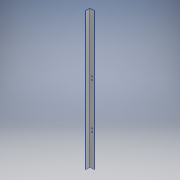
# Autodesk Inventor part: 1400-06-04 Profilé vertical chaniere
Saved by Autodesk Inventor 2017 (Build 210142000, 142)
## iProperties
Part Number: 1400-06-04 Profilé vertical chaniere
Project: 1400-PopCorn Machine
Material: Aluminium 6061
Catalog Web Link: http://www.frenchmakers.com/
Document SubType Name: Modeling
Designer: FABLAB Frenchmakers
Density: 2.7 g/cm^3
Appearance: Aluminium - Plat
Stock Number: 1400-06-03
RuleStatus: InUse
Company: FABLAB Frenchmakers
Author: Adrien MARY
Autodesk Inventor part; units mm, degrees
ref_plane "YZ Plane" through (0, 0, 0) normal (1, 0, 0) x (0, 1, 0)
ref_plane "XZ Plane" through (0, 0, 0) normal (0, 1, 0) x (-1, 0, 0)
ref_plane "XY Plane" through (0, 0, 0) normal (0, 0, 1) x (1, 0, 0)
sketch "Esquisse1" plane through (0, 0, 0) normal (0, 0, 1) x (1, 0, 0)
  line L0 (0, 0) -> (18.3, 0)
  line L1 (18.3, 0) -> (18.3, 2.2)
  line L2 (18.3, 2.2) -> (-2.2, 2.2)
  line L3 (-2.2, 2.2) -> (-2.2, -18.3)
  line L4 (-2.2, -18.3) -> (0, -18.3)
  line L5 (0, -18.3) -> (0, 0)
  dimension "Epaisseur_cornière" = 2.2
  dimension "Largueur" = 20.5
  constraints: 12 end point, 7 perpendicular, 1 horizontal
  measures "Epaisseur_cornière" distance between parallel lines of L2 L0
  measures "Largueur" distance of L1.end L2.end
extrude "Embase" add sketch "Esquisse1" along normal mid plane 610.2
sketch "Esquisse2" plane through (0, 0, 0) normal (0, 1, 0) x (-1, 0, 0)
  line L0 (2.2, 305.1) -> (-18.3, 284.6)
  line L1 (-18.3, 284.6) -> (-18.3, 305.1)
  line L2 (-18.3, 305.1) -> (2.2, 305.1)
  line L3 (-18.3, 305.1) -> (2.2, 305.1) construction
  line L4 (2.2, -305.1) -> (2.2, 305.1) construction
  line L5 (-18.3, -305.1) -> (-18.3, 305.1) construction
  point P0 (0, 0)
  dimension "d4" = 45
  constraints: 6 end point, 2 collinear, 1 vertical
  measures "d4" angle of L1 L0
extrude "Découpe à 45" [suppressed]
mirror "Symétrie découpe" [suppressed]
sketch "Esquisse3" plane through (-2.2, 2.2, 305.1) normal (0, 1, 0) x (1, 0, 0)
  line L0 (0, 610.2) -> (20.5, 610.2) construction
  line L1 (20.5, 610.2) -> (20.5, 0) construction
  line L2 (2.2, 0) -> (2.2, 610.2) construction
  point P0 (2.2, 305.1)
  point P1 (11.35, 470.2)
  point P2 (11.35, 456.2)
  dimension "d7" = 14
  dimension "d8" = 140
  dimension "d9" = 9.15
  dimension "d17" = 18.3
  constraints: 1 vertical alignment
  measures "d7" distance of point (11.35, 456.2) point (11.35, 470.2)
  measures "d8" distance from line of point (11.35, 470.2) L0
  measures "d9" distance from line of L1 point (11.35, 470.2)
  measures "d17" distance between parallel lines of L2 L1
hole "Perçage1" at (9.15, 2.2, -165.1) at (9.15, 2.2, -151.1) direction (0, -1, 0) diameter 5.5 end through all clearance for "Vis à tête plate fraisée ISO 2009/7046" size "M5" standard "ISO"
pattern_linear "Réseau rectangulaire1" count 2 spacing 200 along (0, 0, 1) of "Perçage1"
equation "\"d9\" = 0.5 * d17"
